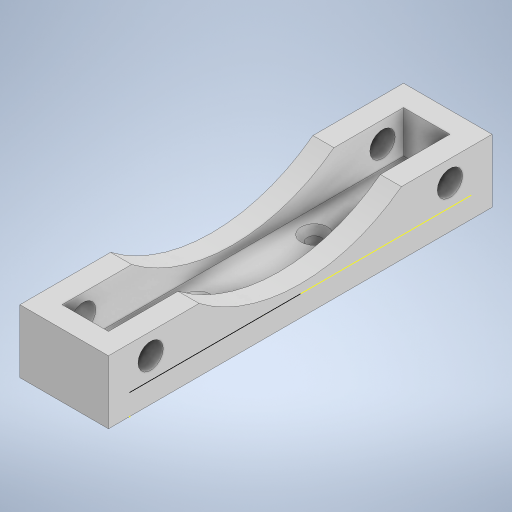
# Autodesk Inventor part: Base ventilador ahora si
Saved by Autodesk Inventor 2024.3 (Build 283343000, 343)
## iProperties
Created: 2025-01-28
Part Number: Base ventilador ahora si
Material: Genérico
Document SubType Name: Modeling
Designer: leivi
Density: 1 g/cm^3
Appearance: Valor por defecto
Author: leivi
Autodesk Inventor part; units mm, degrees
ref_plane "YZ Plane" through (0, 0, 0) normal (1, 0, 0) x (0, 1, 0)
ref_plane "XZ Plane" through (0, 0, 0) normal (0, 1, 0) x (-1, 0, 0)
ref_plane "XY Plane" through (0, 0, 0) normal (0, 0, 1) x (1, 0, 0)
sketch "Boceto1" plane through (0, 0, 0) normal (0, 1, 0) x (-1, 0, 0)
  point P0 (0, 0)
sketch "Boceto2" plane through (0, 0, 0) normal (0, 1, 0) x (-1, 0, 0)
  line L0 (0, 0) -> (11, 0)
  line L1 (11, 0) -> (11, -81)
  line L2 (11, -81) -> (0, -81)
  line L3 (0, -81) -> (0, 0)
  line L4 (-5, 0) -> (-5, 5)
  line L5 (11, -86) -> (16, -86)
  line L6 (-5, 5) -> (16, 5)
  line L7 (16, 5) -> (16, -86)
  line L8 (16, -86) -> (-5, -86)
  line L9 (-5, -86) -> (-5, 5)
  dimension "d0" = 81
  dimension "d1" = 5
  dimension "d2" = 5
  dimension "d3" = 5
  dimension "d4" = 5
  constraints: 20 end point, 4 parallel, 2 horizontal, 2 perpendicular
  measures "d0" distance of L0.end L1.end
  measures "d1" distance of L0.start L4.start
  measures "d2" distance of L4.start L4.end
  measures "d3" distance of L1.end L5.start
  measures "d4" distance of L5.start L5.end
extrude "Extrusión1" add sketch "Boceto2" along normal blind 15
sketch "Boceto3" plane through (0, 0, 0) normal (0, -1, 0) x (1, 0, 0)
  line L0 (0, -81) -> (0, 0) projected
  line L1 (-11, 0) -> (-11, -81) projected
  line L2 (0, 0) -> (-11, 0)
  line L3 (-11, 0) -> (-11, -81)
  line L4 (-11, -81) -> (0, -81)
  line L5 (0, -81) -> (0, 0)
  constraints: 8 end point, 2 parallel, 1 horizontal, 1 perpendicular
extrude "Extrusión2" add sketch "Boceto3" against normal blind 5
sketch "Boceto4" plane through (0, 5, 0) normal (0, 1, 0) x (1, 0, 0)
  line L0 (0, 0) -> (-11, 0) projected
  line L1 (-5.5, 0) -> (-5.5, 81)
  line L2 (-11, 81) -> (0, 81) projected
  line L3 (-5.5, 0) -> (-5.5, 26.66)
  line L4 (-5.5, 81) -> (-5.5, 54.34)
  dimension "d9" = 26.66
  dimension "d10" = 26.66
  constraints: 6 end point, 2 midpoint, 2 point on line
  measures "d9" distance of L1.start L3.end
  measures "d10" distance of L1.end L4.end
hole "Agujero1" at (-5.5, 5, -26.66) at (-5.5, 5, -54.34) direction (0, -1, 0) diameter 3.4 depth 5 countersink diameter 6.3 countersink angle 90 clearance for "Tornillo para maquinaria de cabeza plana" size "M3" standard "Perfil M métrico ANSI"
sketch "Boceto5" plane through (5, 0, 5) normal (1, 0, 0) x (0, 0, -1)
  line L0 (0, 0) -> (45.5, 0)
  line L1 (0, 0) -> (91, 0) projected
  line L2 (45.5, 0) -> (45.5, 5)
  line L3 (45.5, 5) -> (45.5, 7)
  line L4 (45.5, 7) -> (45.5, 47)
  circle A0 centre (45.5, 47) radius 40
  point P0 (5, 0)
  dimension "d18" = 45.5
  dimension "d19" = 5
  dimension "d20" = 2
  dimension "d21" = 40
  constraints: 8 end point, 1 coincident, 1 midpoint, 1 perpendicular, 1 point on line, 1 vertical, 1 vertical alignment, 2 other
  measures "d18" distance of L0.start L0.end
  measures "d19" distance of L0.end L2.end
  measures "d20" distance of L2.end L3.end
  measures "d21" distance of L3.end L4.end
extrude "Extrusión3" cut sketch "Boceto5" against normal blind 32
sketch "Boceto6" plane through (5, 0, 5) normal (1, 0, 0) x (0, 0, -1)
  line L0 (0, 0) -> (0, 15) projected
  line L1 (91, 0) -> (91, 15) projected
  line L2 (91, 0) -> (0, 0) projected
  line L3 (0, 0) -> (10, 0)
  line L4 (10, 0) -> (10, 10)
  circle A0 centre (10, 10) radius 3
  line L5 (91, 0) -> (81, 0)
  line L6 (0, 0) -> (91, 0) projected
  line L7 (81, 0) -> (81, 10)
  circle A1 centre (81, 10) radius 3
  point P0 (5, 0)
  dimension "d26" = 10
  dimension "d27" = 10
  dimension "d29" = 6
  dimension "d30" = 10
  dimension "d31" = 10
  constraints: 8 end point, 2 centre point, 2 coincident, 2 perpendicular, 2 point on line
  measures "d26" distance of L0.start L3.end
  measures "d27" distance of L3.end L4.end
  measures "d29" diameter of A0
  measures "d30" distance of L1.start L5.end
  measures "d31" distance of L5.end L7.end
sketch "Boceto7" plane through (5, 0, 5) normal (1, 0, 0) x (0, 0, -1)
  line L0 (5, 5) -> (45.5, 5)
  line L1 (86, 5) -> (5, 5) projected
  point P0 (5, 0)
  constraints: 2 end point, 1 midpoint
extrude "Extrusión4" cut sketch "Boceto6" against normal blind 58
